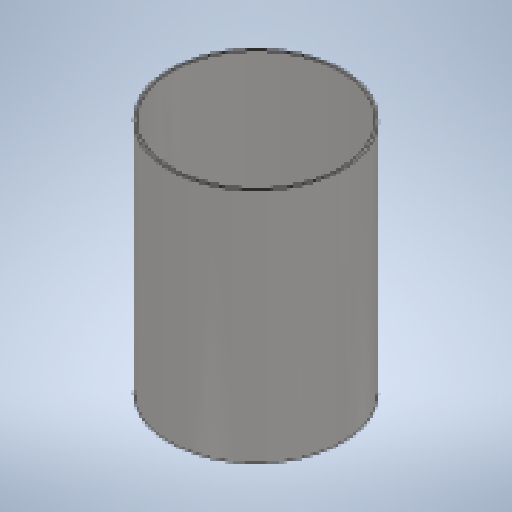
# Autodesk Inventor part: TKS 3102 TOP DS main tube
Saved by Autodesk Inventor 2025.1 (Build 291241020, 241B)
## iProperties
Created: 2025-02-19
Part Number: TKS 3102 TOP DS main tube
Material: Stainless Steel
Document SubType Name: Modeling
Designer: user
Density: 8 g/cm^3
Appearance: Semi-Polished
Author: admin
Autodesk Inventor part; units mm, degrees
ref_plane "YZ Plane" through (0, 0, 0) normal (1, 0, 0) x (0, 1, 0)
ref_plane "XZ Plane" through (0, 0, 0) normal (0, 1, 0) x (-1, 0, 0)
ref_plane "XY Plane" through (0, 0, 0) normal (0, 0, 1) x (1, 0, 0)
sketch "Sketch1" plane through (0, 0, 0) normal (0, 0, 1) x (1, 0, 0)
  circle A0 centre (0, 0) radius 110
  circle A1 centre (0, 0) radius 107
  dimension "d0" = 220
  dimension "d1" = 3
  constraints: 2 centre point, 1 coincident
  measures "d0" diameter of A0
  measures "d1" radial gap between concentric circles of A0 A1
extrude "Extrusion1" add sketch "Sketch1" along normal blind 300
body "Solid1"
